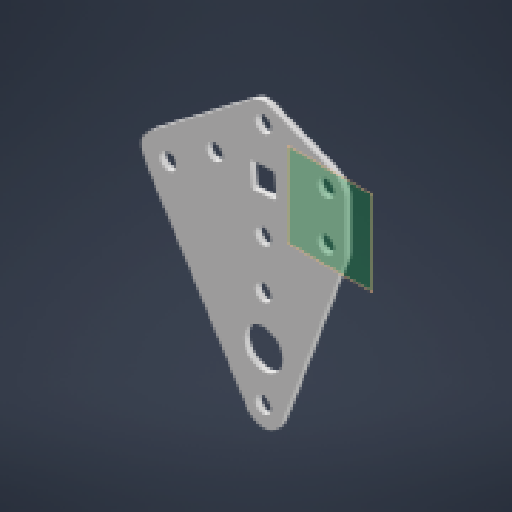
# Autodesk Inventor part: inner-pto-shaft-support
Saved by Autodesk Inventor 2023.2 (Build 272271000, 271)
## iProperties
Created: 2023-03-20
Part Number: inner-pto-shaft-support
Material: Generic
Document SubType Name: Modeling
Designer: Liam
Density: 1 g/cm^3
Appearance: Default
Author: Liam
Autodesk Inventor part; units mm, degrees
ref_plane "YZ Plane" through (0, 0, 0) normal (1, 0, 0) x (0, 1, 0)
ref_plane "XZ Plane" through (0, 0, 0) normal (0, 1, 0) x (-1, 0, 0)
ref_plane "XY Plane" through (0, 0, 0) normal (0, 0, 1) x (1, 0, 0)
ref_plane "Work Plane2" through (0, 0, 0) normal (0, 0, -1) x (-1, 0, 0)
sketch "Sketch2" plane through (0, 0, 0) normal (0, 0, -1) x (-1, 0, 0)
  line L0 (45.0497, -16.3832) -> (21.7462, -53.5011)
  arc A0 (12.6742, -52.5484) -> (21.7462, -53.5011) centre (17.4439, -50.8) ccw
  line L1 (12.6742, -52.5484) -> (-3.6199, -8.0984)
  circle A1 centre (17.4439, -38.1) radius 5
  circle A2 centre (17.4439, -25.4) radius 2.1082
  circle A3 centre (17.4439, -12.7) radius 2.1082
  circle A4 centre (30.1439, 0) radius 2.1082
  circle A5 centre (17.4439, 12.7) radius 2.1082
  line L2 (-0.6948, 11.0833) -> (15.5993, 17.4333)
  arc A6 (-0.6948, 11.0833) -> (-3.9302, 6.35) centre (1.1498, 6.35) ccw
  arc A7 (-3.9302, -6.35) -> (-3.6199, -8.0984) centre (1.1498, -6.35) ccw
  line L3 (-3.9302, -6.35) -> (-3.9302, 6.35)
  circle A8 centre (1.1498, 6.35) radius 2.1844
  circle A9 centre (1.1498, -6.35) radius 2.1844
  circle A10 centre (42.2678, -8.0984) radius 2.0955
  circle A11 centre (17.4439, -50.8) radius 2.0955
  line L4 (21.036, 16.2921) -> (46.2505, -3.0363)
  spline S0 degree 4 poles (15.5993, 17.4333) (16.2989, 17.7059) (17.6982, 18.2512) (19.3014, 17.6218) (20.4578, 16.7353) (21.036, 16.2921) knots 0 0 0 0 0 0.5 1 1 1 1 1
  spline S1 degree 4 poles (46.2505, -3.0363) (47.8892, -4.2924) (51.1665, -6.8047) (47.8672, -11.8956) (45.9889, -14.8873) (45.0497, -16.3832) knots 0 0 0 0 0 0.5 1 1 1 1 1
  arc A12 (20.8415, 2.2589) -> (20.2651, 2.9475) centre (20.209, 2.315) ccw projected
  line L5 (20.2651, 2.9475) -> (15.185, 3.3976) projected
  arc A13 (15.185, 3.3976) -> (14.4964, 2.8212) centre (15.1289, 2.7651) ccw projected
  line L6 (14.4964, 2.8212) -> (14.0462, -2.2589) projected
  arc A14 (14.0462, -2.2589) -> (14.6227, -2.9475) centre (14.6788, -2.315) ccw projected
  line L7 (14.6227, -2.9475) -> (19.7028, -3.3976) projected
  arc A15 (19.7028, -3.3976) -> (20.3914, -2.8212) centre (19.7589, -2.7651) ccw projected
  line L8 (20.3914, -2.8212) -> (20.8415, 2.2589) projected
  point P0 (0, 0)
  dimension "d37" = 10
  dimension "d38" = 4.191
  dimension "d39" = 4.2164
  dimension "d40" = 4.2164
  dimension "d41" = 4.2164
  dimension "d42" = 4.3688
  dimension "d43" = 4.3688
  dimension "d44" = 4.191
  constraints: 12 centre point, 10 end point, 6 point on circle, 1 coincident, 1 tangent, 19 other
  measures "d37" diameter of A1
  measures "d38" diameter of A11
  measures "d39" diameter of A2
  measures "d40" diameter of A3
  measures "d41" diameter of A4
  measures "d42" diameter of A8
  measures "d43" diameter of A9
  measures "d44" diameter of A10
extrude "Extrusion3" add sketch "Sketch2" along normal blind 1.524
body "Solid2"
